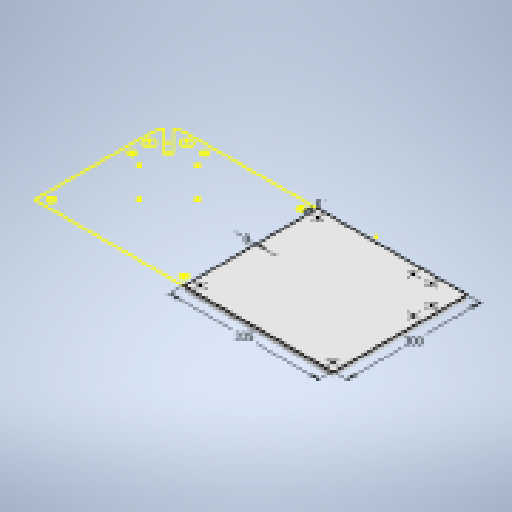
# Autodesk Inventor part: Right top plate
Saved by Autodesk Inventor 2024 (Build 280153000, 153)
## iProperties
Created: 2024-03-26
Part Number: Right top plate
Material: Generic
Document SubType Name: Modeling
Designer: jens1
Density: 1 g/cm^3
Appearance: Default
Author: jens1
Autodesk Inventor part; units mm, degrees
ref_plane "YZ Plane" through (0, 0, 0) normal (1, 0, 0) x (0, 1, 0)
ref_plane "XZ Plane" through (0, 0, 0) normal (0, 1, 0) x (-1, 0, 0)
ref_plane "XY Plane" through (0, 0, 0) normal (0, 0, 1) x (1, 0, 0)
sketch "Sketch1" plane through (0, 0, 0) normal (0, 1, 0) x (-1, 0, 0)
  circle A0 centre (275.1702, 127.184) radius 4.5 projected
  circle A1 centre (341.1702, 61.184) radius 4.5 projected
  circle A2 centre (341.1702, 193.184) radius 4.5 projected
  circle A3 centre (407.1702, 127.184) radius 4.5 projected
  line L0 (404.6478, 74.313) -> (450.2561, 28.7046) projected
  arc A4 (450.2561, 28.7046) -> (457.1702, 51.184) centre (417.1702, 51.184) ccw projected
  line L1 (457.1702, 51.184) -> (457.1702, 311.184) projected
  line L2 (457.1702, 311.184) -> (122.1702, 311.184) projected
  line L3 (122.1702, 311.184) -> (122.1702, 11.184) projected
  line L4 (122.1702, 11.184) -> (417.1702, 11.184) projected
  arc A5 (417.1702, 11.184) -> (439.6495, 18.098) centre (417.1702, 51.184) ccw projected
  line L5 (439.6495, 18.098) -> (394.0412, 63.7064) projected
  arc A6 (404.6478, 74.313) -> (394.0412, 63.7064) centre (399.3445, 69.0097) ccw projected
  circle A7 centre (438.3202, 72.034) radius 11.75 projected
  circle A8 centre (396.3202, 30.034) radius 11.75 projected
  circle A9 centre (356.7202, 30.034) radius 7.85 projected
  circle A10 centre (438.3202, 111.634) radius 7.85 projected
  circle A11 centre (141.0202, 292.334) radius 7.85 projected
  circle A12 centre (141.0202, 30.034) radius 7.85 projected
  circle A13 centre (438.3202, 292.334) radius 7.85 projected
  line L6 (122.1702, 11.184) -> (-212.8298, 11.184)
  line L7 (-212.8298, 11.184) -> (-212.8298, 311.184)
  line L8 (-212.8298, 311.184) -> (122.1702, 311.184)
  line L9 (122.1702, 311.184) -> (122.1702, 11.184)
  point P0 (0, 0)
  point P1 (-193.9798, 72.034)
  point P2 (-151.9798, 30.034)
  point P3 (-112.3798, 30.034)
  point P4 (-193.9798, 111.634)
  point P5 (103.3202, 292.334)
  point P6 (103.3202, 30.034)
  point P7 (-193.9798, 292.334)
  point P8 (103.3202, 292.334)
  point P9 (103.3202, 30.034)
  point P10 (-112.3798, 30.034)
  point P11 (-151.9798, 30.034)
  point P12 (-193.9798, 72.034)
  point P13 (-193.9798, 111.634)
  point P14 (-193.9798, 292.334)
  dimension "d0" = 335
  dimension "d1" = 300
  dimension "d2" = 0
  dimension "d3" = 0
  constraints: 8 end point, 7 coincident, 7 symmetric about line, 2 parallel, 1 horizontal, 1 perpendicular
  measures "d0" distance of L7.end L8.end
  measures "d1" distance of L6.end L7.end
  measures "d2" distance between parallel lines of L3 L9
  measures "d3" distance between parallel lines of L4 L6
extrude "Extrusion1" add sketch "Sketch1" against normal blind 10.5 contours L3 L6 L7 L8
hole "Hole2" at (-103.3202, 0, 292.334) at (-103.3202, 0, 30.034) at (112.3798, 0, 30.034) at (193.9798, 0, 111.634) at (193.9798, 0, 292.334) direction (0, -1, 0) diameter 8 end through all countersink diameter 15.7 countersink angle 90
hole "Hole3" at (151.9798, 0, 30.034) at (193.9798, 0, 72.034) direction (0, -1, 0) diameter 12 end through all countersink diameter 23.5 countersink angle 90
fillet "Fillet1" radius 40 1 edges at (212.8298, -5.25, 11.184)
body "Solid1"
